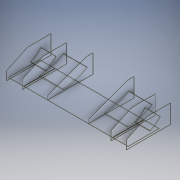
# Autodesk Inventor part: F-wing
Saved by Autodesk Inventor 2018.1 (Build 221171000, 171)
## iProperties
Created: 2017-10-11
Part Number: F-wing
Material: CFRP
Document SubType Name: Modeling
Designer: kuwano
Density: 1.43 g/cm^3
Appearance: カーボンファイバー 1
Mass: 9300.44 g
Surface Area: 23786.1 cm^2
Volume: 6503.8 cm^3
Author: kuwano
Autodesk Inventor part; units mm, degrees
sketch "スケッチ1" plane through (0, 0, 0) normal (1, 0, 0) x (0, 1, 0)
  line L0 (5, 175) -> (0, 175)
  line L1 (0, 175) -> (0, -175)
  line L2 (0, -175) -> (5, -175)
  line L3 (5, -175) -> (5, 175)
  point P0 (0, 0)
  dimension "d0" = 350
  dimension "d1" = 5
  constraints: 8 end point, 2 midpoint, 2 parallel, 1 horizontal, 1 perpendicular
  measures "d0" distance of L0.end L1.end
  measures "d1" distance of L1.end L2.end
extrude "押し出し1" add sketch "スケッチ1" along normal mid plane 1350
sketch "スケッチ2" plane through (675, 0, 0) normal (1, 0, 0) x (0, 0, -1)
  line L0 (40.8958, 190) -> (-195, 80)
  line L1 (-195, 80) -> (-195, -20)
  line L2 (-195, -20) -> (305, -20)
  line L3 (305, -20) -> (305, 190)
  line L4 (-175, 0) -> (175, 0) projected
  line L5 (-175, 5) -> (-175, 0) projected
  line L6 (175, 0) -> (175, 5) projected
  line L7 (175, 5) -> (-175, 5) projected
  line L8 (40.8958, 190) -> (305, 190)
  point P0 (0, 0)
  dimension "d4" = 20
  dimension "d5" = 25
  dimension "d6" = 210
  dimension "d7" = 500
  dimension "d8" = 20
  dimension "d9" = 100
  constraints: 10 end point, 3 parallel, 1 horizontal
  measures "d4" distance between parallel lines of L2 L4
  measures "d5" angle of L7 L0
  measures "d6" distance of L2.end L3.end
  measures "d7" distance of L1.end L2.end
  measures "d8" distance between parallel lines of L5 L1
  measures "d9" distance of L0.end L1.end
extrude "押し出し3" add sketch "スケッチ2" along normal blind 3 contours L8 L3 L2 L1 L0 | L5 L7 L6 L4
ref_plane "作業平面1" through (230, 0, 0) normal (1, 0, 0) x (0, 1, 0)
ref_plane "作業平面2" through (589, 0, 0) normal (-1, 0, 0) x (0, 0, 1)
ref_plane "作業平面3" through (230, 0, 0) normal (1, 0, 0) x (0, 1, 0)
mirror "ミラー3" about plane through (589, 0, 0) normal (-1, 0, 0) of "押し出し3"
sketch "スケッチ4" plane through (230, 0, 0) normal (1, 0, 0) x (0, 1, 0)
  line L0 (50, 175) -> (0, 175)
  line L1 (0, 175) -> (0, -335)
  line L2 (0, -335) -> (210, -335)
  line L3 (210, -335) -> (210, -264.5964)
  line L4 (210, -264.5964) -> (50, 175)
  line L5 (0, -561) -> (0, 321) projected
  line L6 (80, 195) -> (-20, 195) projected
  line L7 (-20, 195) -> (-20, -305) projected
  line L8 (-20, -305) -> (190, -305) projected
  line L9 (190, -305) -> (190, -40.8958) projected
  line L10 (5, 175) -> (0, 175) projected
  point P0 (0, 0)
  dimension "d28" = 30
  dimension "d29" = 20
  dimension "d30" = 50
  dimension "d44" = 20
  constraints: 10 end point, 3 collinear, 1 horizontal, 1 parallel, 1 perpendicular
  measures "d28" distance between parallel lines of L2 L8
  measures "d29" angle of L1 L4
  measures "d30" distance of L0.start L0.end
  measures "d44" distance between parallel lines of L9 L3
extrude "押し出し5" add sketch "スケッチ4" along normal blind 3 contours L4 L9 L8 L1 L0 | L4 L3 L2 L1 L8 L9
sketch "スケッチ5" plane through (675, 0, 0) normal (-1, 0, 0) x (0, 0, 1)
  arc A0 (-205, 136.0374) -> (-25, 10) centre (185.8126, 502.6236) ccw
  line L0 (175, 5) -> (-175, 5) projected
  line L1 (-175, 5) -> (-175, 0) projected
  arc A1 (-205, 136.0374) -> (-25, 10) centre (17.5441, 262.3112) ccw
  line L2 (-25, 10) -> (-205, 136.0374)
  line L3 (-305, -20) -> (-305, 190) projected
  line L4 (-175, 5) -> (175, 5) projected
  point P0 (0, 0)
  dimension "d36" = 5
  dimension "d37" = 150
  dimension "d53" = 35
  dimension "d54" = 100
  constraints: 4 point on circle, 2 centre point, 2 end point
  measures "d36" distance from line of L2.start L0
  measures "d37" distance from line of L2.start L1
  measures "d53" angle of L0 L2
  measures "d54" distance from line of L3 L2.end
extrude "押し出し6" add sketch "スケッチ5" along normal up to next contours A0 A1
sketch "スケッチ6" plane through (500, -20, -305) normal (-1, 0, 0) x (0, 0, 1)
  arc A0 (0, 141.8207) -> (380, 40) centre (380, 800) ccw
  arc A1 (0, 141.8207) -> (380, 40) centre (303.2883, 513.7079) ccw
  line L0 (0, 141.8207) -> (380, 40)
  line L1 (480, 25) -> (130, 25) projected
  line L2 (480, 20) -> (480, 25) projected
  line L3 (380, 40) -> (470.3272, 40)
  line L4 (0, 0) -> (0, 210) projected
  point P0 (305, 20)
  dimension "d45" = 15
  dimension "d46" = 100
  dimension "d48" = 15
  constraints: 4 end point, 4 point on circle, 2 centre point, 1 horizontal, 1 point on line, 1 tangent
  measures "d45" angle of L1 L0
  measures "d46" distance from line of L2 L0.end
  measures "d48" distance between parallel lines of L3 L1
extrude "押し出し7" add sketch "スケッチ6" along normal up to next contours A0 A1
fillet "フィレット2" radius 5 2 edges at (366.5, 20, 75) (589, 10, -25)
fillet "フィレット3" radius 3 2 edges at (366.5, 121.8207, -305) (589, 136.0374, -205)
mirror "ミラー9" about plane through (0, 0, 0) normal (1, 0, 0) of "押し出し5", "押し出し7", "押し出し3", "ミラー3", "押し出し6", "フィレット2", "フィレット3"
